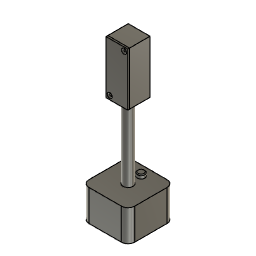
attiny85-traffic-light (Autodesk Fusion 360 design; units mm, degrees)
Autodesk Fusion 360 part; units mm, degrees
note: some values were not read from the file. Set by a fixed rule: which sketch regions a step uses.
sketch "Sketch1" plane through (0, 0, 0) normal (0, 1, 0) x (1, 0, 0)
  line L0 (0, 0) -> (17.5, 0)
  line L1 (17.5, 0) -> (17.5, -42.6)
  line L2 (17.5, -42.6) -> (0, -42.6)
  line L3 (0, -42.6) -> (0, 0)
  circle A0 centre (8.75, -21.3) radius 4.9
  line L4 (0, -21.3) -> (17.5, -21.3) construction
  circle A1 centre (8.75, -33.85) radius 4.9
  circle A2 centre (8.75, -8.75) radius 4.9
  line L5 (1.44, -1.44) -> (16.06, -1.44)
  line L6 (16.06, -1.44) -> (16.06, -41.16)
  line L7 (16.06, -41.16) -> (1.44, -41.16)
  line L8 (1.44, -41.16) -> (1.44, -1.44)
  circle A3 centre (14.5, -39.6) radius 3
  line L9 (11.5, -39.6) -> (11.5, -42.6)
  line L10 (14.5, -36.6) -> (17.5, -36.6)
  circle A4 centre (14.5, -39.6) radius 1.25
  circle A5 centre (3, -3) radius 3
  line L11 (6, -3) -> (6, 0)
  line L12 (3, -6) -> (0, -6)
  circle A6 centre (3, -3) radius 1.25
  circle A7 centre (14.5, -39.6) radius 1
  circle A8 centre (3, -3) radius 1
  line L13 (1.64, -1.64) -> (15.86, -1.64)
  line L14 (15.86, -1.64) -> (15.86, -40.96)
  line L15 (15.86, -40.96) -> (1.64, -40.96)
  line L16 (1.64, -40.96) -> (1.64, -1.64)
  dimension "d4" = 17.5
  dimension "d5" = 42.6
  dimension "d6" = 9.8
  dimension "d9" = 0
  dimension "d10" = 12.55
  dimension "d14" = 1.44
  dimension "d22" = 3
  dimension "d23" = 2.5
  dimension "d24" = 3
  dimension "d25" = 2.5
  dimension "d31" = 2
  dimension "d32" = 2
  dimension "d37" = 1.64
  constraint horizontal L0
  constraint vertical L1
  constraint horizontal L2
  constraint vertical L3
  constraint coincident L0.start L3.end
  constraint midpoint L3 L4.start
  constraint midpoint L1 L4.end
  constraint midpoint A0.centre L4
  constraint tangent L2 A3
  constraint tangent L1 A3
  constraint coincident A3 L9.start
  constraint coincident L2 L9.end
  constraint tangent A3 L9
  constraint perpendicular L2 L9
  constraint coincident A3 L10.start
  constraint coincident L1 L10.end
  constraint tangent A3 L10
  constraint perpendicular L1 L10
  constraint concentric A3 A4
  constraint tangent L3 A5
  constraint tangent L0 A5
  constraint coincident A5 L11.start
  constraint coincident L0 L11.end
  constraint tangent A5 L11
  constraint perpendicular L0 L11
  constraint coincident A5 L12.start
  constraint coincident L3 L12.end
  constraint tangent A5 L12
  constraint perpendicular L3 L12
  constraint concentric A5 A6
  constraint concentric A3 A7
  constraint concentric A6 A8
  measures "d4" distance of L0.start L0.end
  measures "d5" distance of L0.start L2.end
  measures "d6" diameter of A0
  measures "d22" radius of A3
  measures "d23" diameter of A4
  measures "d24" radius of A5
  measures "d25" diameter of A6
  measures "d31" diameter of A7
  measures "d32" diameter of A8
extrude "Extrude1" add sketch "Sketch1" along normal blind 4.44 contours L0 L5 A5 L11 | L0 L1 L5 L6 L10 L11 | L0 L3 A5 | L5 L8 A5 | L5 A5 L11 L13 | L5 L6 L10 L11 L13 L14 | L1 L6 A3 L10 | L5 L8 A5 L13 L16 | L3 L8 A5 L12 | A3 L9 L10 A5 L11 L12 L13 L14 L15 L16 | A5 L11 L13 | L6 L7 A3 | L1 L2 A3 | L6 A3 L10 L14 | A5 L13 L16 | L2 L3 L7 L8 L9 L12 | L8 A5 L12 L16 | L6 L7 A3 L14 L15 | L2 L7 A3 L9 | A3 L10 L14 | L7 L8 L9 L12 L15 L16 | A5 L12 L16 | A3 L14 L15 | L7 A3 L9 L15 | A3 L9 L15 | A4 | A6 | A7 | A8 makes body 1
extrude "Extrude2" add sketch "Sketch1" against normal blind 12.06 separate body contours L0 L5 A5 L11 | L0 L1 L5 L6 L10 L11 | L0 L3 A5 | L5 L8 A5 | L1 L6 A3 L10 | L3 L8 A5 L12 | L6 L7 A3 | L1 L2 A3 | L2 L3 L7 L8 L9 L12 | L2 L7 A3 L9 makes body 2
extrude "Extrude3" add sketch "Sketch1" against normal blind 11.26 separate body contours L5 A5 L11 L13 | L5 L8 A5 L13 L16 | A5 L11 L13 | L6 A3 L10 L14 | A5 L13 L16 | L8 A5 L12 L16 | L6 L7 A3 L14 L15 | A3 L10 L14 | A5 L12 L16 | A3 L14 L15 | L7 A3 L9 L15 | A3 L9 L15 makes body 3 at (13.3254, -7.5067, 40.0275) makes body 4 at (4.2438, -3.7533, 3.1245)
combine "Combine1" operation add target body 2 tool bodies 3 4
combine "Combine2" operation add target body 1 tool bodies 2
extrude "Extrude4" add sketch "Sketch1" against normal blind 1.44 from surface at -12.06 separate body contours L0 L5 A5 L11 | L0 L1 L5 L6 L10 L11 | L0 L3 A5 | L5 L8 A5 | L5 A5 L11 L13 | L5 L6 L10 L11 L13 L14 | L1 L6 A3 L10 | L5 L8 A5 L13 L16 | L3 L8 A5 L12 | A3 L9 L10 A5 L11 L12 L13 L14 L15 L16 | A5 L11 L13 | L6 L7 A3 | L1 L2 A3 | L6 A3 L10 L14 | A5 L13 L16 | L2 L3 L7 L8 L9 L12 | L8 A5 L12 L16 | L6 L7 A3 L14 L15 | L2 L7 A3 L9 | A3 L10 L14 | L7 L8 L9 L12 L15 L16 | A5 L12 L16 | A3 L14 L15 | L7 A3 L9 L15 | A3 L9 L15 | A0 | A1 | A2 | A4 | A6 makes body 5
extrude "Extrude5" add sketch "Sketch1" along normal blind 0.6 from surface at -12.06 contours A3 L9 L10 A5 L11 L12 L13 L14 L15 L16 | A5 L11 L13 | A5 L13 L16 | A3 L10 L14 | A5 L12 L16 | A3 L14 L15 | A3 L9 L15 | A0 | A1 | A2 | A4 | A6 bodies 5
chamfer "Chamfer1" distance 1 angle 45 2 edges at (13.5677, -13.5, 39.9616) (2.0677, -13.5, 3.3616) on bodies 5
sketch "Sketch2" plane through (0, 0, 0) normal (0, 0, 1) x (1, 0, 0)
  circle A0 centre (8.75, -4.53) radius 3
  line L0 (0, 0) -> (17.5, 0)
  line L1 (17.5, 0) -> (17.5, 4.44)
  line L2 (17.5, 4.44) -> (0, 4.44)
  line L3 (0, 4.44) -> (0, 0)
  line L4 (0, 0) -> (17.5, 0)
  line L5 (17.5, 0) -> (17.5, -13.5)
  line L6 (17.5, -13.5) -> (0, -13.5)
  line L7 (0, -13.5) -> (0, 0)
  line L8 (8.75, 4.44) -> (8.75, -13.5)
  circle A1 centre (8.75, -4.53) radius 4
  circle A2 centre (8.75, -4.53) radius 3.8
  line L9 (8.75, -0.53) -> (8.95, -0.53)
  line L10 (8.95, -0.53) -> (8.95, -8.53)
  line L11 (8.95, -8.53) -> (8.75, -8.53)
  line L12 (8.75, -8.53) -> (8.75, -0.53)
  line L13 (8.75, -0.53) -> (8.55, -0.53)
  line L14 (8.55, -0.53) -> (8.55, -8.53)
  line L15 (8.55, -8.53) -> (8.75, -8.53)
  line L16 (8.75, -8.53) -> (8.75, -0.53)
  line L17 (8.75, -4.53) -> (4.75, -4.53)
  line L18 (8.75, -4.53) -> (12.75, -4.53)
  line L19 (12.75, -4.63) -> (4.75, -4.63)
  line L20 (4.75, -4.63) -> (4.75, -4.43)
  line L21 (4.75, -4.43) -> (12.75, -4.43)
  line L22 (12.75, -4.43) -> (12.75, -4.63)
  line L23 (12.75, -4.63) -> (4.75, -4.43) construction
  line L24 (4.75, -4.63) -> (12.75, -4.43) construction
  point P0 (8.75, -4.53)
  dimension "d41" = 6
  dimension "d42" = 17.5
  dimension "d43" = 4.44
  dimension "d44" = 17.5
  dimension "d45" = 13.5
  dimension "d46" = 1
  dimension "d52" = 0.8
  dimension "d53" = 0.2
  dimension "d54" = 8
  dimension "d124" = 0.2
  dimension "d125" = 8
  dimension "d126" = 8
  dimension "d127" = 0.2
  constraint horizontal L0
  constraint vertical L1
  constraint horizontal L2
  constraint vertical L3
  constraint coincident L0.start L3.end
  constraint horizontal L4
  constraint vertical L5
  constraint horizontal L6
  constraint vertical L7
  constraint midpoint L2 L8.start
  constraint midpoint L6 L8.end
  constraint midpoint P0 L8
  constraint horizontal L9
  constraint vertical L10
  constraint horizontal L11
  constraint vertical L12
  constraint coincident L8 L9.start
  constraint coincident A1 L9.start
  constraint horizontal L13
  constraint vertical L14
  constraint horizontal L15
  constraint vertical L16
  constraint coincident P0 A0.centre
  constraint coincident A1 L17.end
  constraint horizontal L17
  constraint coincident A1 L18.end
  constraint parallel L17 L18
  constraint horizontal L19
  constraint perpendicular L19 L20
  constraint parallel L19 L21
  constraint parallel L20 L22
  constraint coincident L23 P0
  constraint coincident L24 P0
  measures "d41" diameter of A0
  measures "d42" distance of L0.start L0.end
  measures "d43" distance of L0.start L2.end
  measures "d44" distance of L0.start L0.end
  measures "d45" distance of L0.start L6.end
  measures "d53" distance of L9.start L9.end
  measures "d54" distance of L9.start L11.end
  measures "d124" distance of L9.start L13.end
  measures "d125" distance of L9.start L11.end
  measures "d126" distance of L20.end L21.end
  measures "d127" distance of L19.end L20.end
extrude "Extrude6" add sketch "Sketch2" against normal blind 60 separate body contours A0 A2 L18 L19 | A0 A2 L18 L21 | A0 A2 L10 L21 | A0 A2 L10 L19 | A1 A2 L18 L19 L22 | A1 A2 L18 L21 L22 | A0 L8 A2 L10 L12 L16 | A1 A2 L10 L21 | A0 L8 A2 L10 L12 L16 | A1 A2 L10 L19 | A0 L8 A2 L12 L14 L16 | L8 A1 A2 L10 L12 L16 | A0 L8 A2 L12 L14 L16 | L8 A1 A2 L10 L12 L16 | A0 A2 L14 L21 | L8 A1 A2 L12 L14 L16 | A0 A2 L14 L19 | L8 A1 A2 L12 L14 L16 | A0 A2 L17 L21 | A0 A2 L17 L19 | A1 A2 L14 L21 | A1 A2 L14 L19 | A1 A2 L17 L20 L21 | A1 A2 L17 L19 L20 makes body 6
extrude "Extrude7" cut sketch "Sketch2" along normal blind 1.44 contours A0 L10 L18 L21 | A0 A2 L18 L19 | A0 A2 L18 L21 | A0 L10 L18 L19 | A0 L10 L21 | A0 A2 L10 L21 | A0 A2 L10 L19 | A0 L10 L19 | A1 A2 L18 L19 L22 | A1 A2 L18 L21 L22 | L8 L10 L12 L16 L18 L21 | L8 L10 L12 L16 L18 L19 | A0 L8 L10 L12 L16 L21 | A0 L8 A2 L10 L12 L16 | A1 A2 L10 L21 | A0 L8 A2 L10 L12 L16 | A0 L8 L10 L12 L16 L19 | A1 A2 L10 L19 | L8 L12 L14 L16 L17 L21 | L8 L12 L14 L16 L17 L19 | A0 L8 L12 L14 L16 L21 | L8 A1 A2 L10 L12 L16 | A0 L8 L12 L14 L16 L19 | L8 A1 A2 L10 L12 L16 | A0 L14 L17 L21 | A0 L14 L17 L19 | A0 L14 L21 | A0 L14 L19 bodies 1
extrude "Extrude8" add sketch "Sketch2" along normal blind 1.8 contours A0 A2 L18 L19 | A0 A2 L18 L21 | A0 A2 L10 L21 | A0 A2 L10 L19 bodies 6
ref_plane "WorkPlane1" through (0, 0, -83.68) normal (0, 0, 1) x (1, 0, 0)
sketch "Sketch3" plane through (0, 0, -83.68) normal (0, 0, 1) x (1, 0, 0)
  line L0 (0, 0) -> (8.75, 0) construction
  line L1 (8.75, 0) -> (8.75, -4.53) construction
  line L2 (8.75, -4.53) -> (0, -4.53) construction
  line L3 (0, -4.53) -> (0, 0) construction
  line L4 (21.75, 12.47) -> (-4.25, 12.47)
  line L5 (-8.25, 8.47) -> (-8.25, -17.53)
  line L6 (-4.25, -21.53) -> (21.75, -21.53)
  line L7 (25.75, -17.53) -> (25.75, 8.47)
  line L8 (25.75, 12.47) -> (-8.25, -21.53) construction
  line L9 (-8.25, 12.47) -> (25.75, -21.53) construction
  arc A0 (-8.25, -17.53) -> (-4.25, -21.53) centre (-4.25, -17.53) ccw
  arc A1 (21.75, -21.53) -> (25.75, -17.53) centre (21.75, -17.53) ccw
  arc A2 (25.75, 8.47) -> (21.75, 12.47) centre (21.75, 8.47) ccw
  arc A3 (-4.25, 12.47) -> (-8.25, 8.47) centre (-4.25, 8.47) ccw
  line L10 (-9.69, 8.47) -> (-9.69, -17.53)
  arc A4 (-9.69, -17.53) -> (-4.25, -22.97) centre (-4.25, -17.53) ccw
  line L11 (-4.25, -22.97) -> (21.75, -22.97)
  arc A5 (21.75, -22.97) -> (27.19, -17.53) centre (21.75, -17.53) ccw
  line L12 (27.19, -17.53) -> (27.19, 8.47)
  arc A6 (27.19, 8.47) -> (21.75, 13.91) centre (21.75, 8.47) ccw
  line L13 (21.75, 13.91) -> (-4.25, 13.91)
  arc A7 (-4.25, 13.91) -> (-9.69, 8.47) centre (-4.25, 8.47) ccw
  line L14 (-8.05, 8.47) -> (-8.05, -17.53)
  arc A8 (-8.05, -17.53) -> (-4.25, -21.33) centre (-4.25, -17.53) ccw
  line L15 (-4.25, -21.33) -> (21.75, -21.33)
  arc A9 (21.75, -21.33) -> (25.55, -17.53) centre (21.75, -17.53) ccw
  line L16 (25.55, -17.53) -> (25.55, 8.47)
  arc A10 (25.55, 8.47) -> (21.75, 12.27) centre (21.75, 8.47) ccw
  line L17 (21.75, 12.27) -> (-4.25, 12.27)
  arc A11 (-4.25, 12.27) -> (-8.05, 8.47) centre (-4.25, 8.47) ccw
  line L18 (25.75, -4.53) -> (-8.25, -4.53) construction
  line L19 (8.75, -4.53) -> (12.75, -4.53) construction
  circle A12 centre (12.75, -4.53) radius 11
  line L20 (8.75, -4.53) -> (-3.25, -4.53) construction
  line L21 (-0.25, -14.53) -> (-6.25, -14.53)
  line L22 (-6.25, -14.53) -> (-6.25, 5.47)
  line L23 (-6.25, 5.47) -> (-0.25, 5.47)
  line L24 (-0.25, 5.47) -> (-0.25, -14.53)
  line L25 (-0.25, -14.53) -> (-6.25, 5.47) construction
  line L26 (-6.25, -14.53) -> (-0.25, 5.47) construction
  line L27 (-6.25, -10.43) -> (-0.25, -10.43)
  line L28 (-0.25, -10.43) -> (-0.25, 1.37)
  line L29 (-0.25, 1.37) -> (-6.25, 1.37)
  line L30 (-6.25, 1.37) -> (-6.25, -10.43)
  line L31 (-6.25, -10.43) -> (-0.25, 1.37) construction
  line L32 (-0.25, -10.43) -> (-6.25, 1.37) construction
  line L33 (1.75, -15.53) -> (23.75, -15.53) construction
  line L34 (23.75, -15.53) -> (23.75, 6.47) construction
  line L35 (23.75, 6.47) -> (1.75, 6.47) construction
  line L36 (1.75, 6.47) -> (1.75, -15.53) construction
  line L37 (1.75, -15.53) -> (23.75, 6.47) construction
  line L38 (23.75, -15.53) -> (1.75, 6.47) construction
  line L39 (4.9718, 3.2482) -> (8.1937, 6.47) construction
  circle A13 centre (3.6373, 4.5827) radius 1.8873 construction
  line L40 (4.9718, -12.3082) -> (8.1937, -15.53) construction
  circle A14 centre (3.6373, -13.6427) radius 1.8873 construction
  circle A15 centre (12.75, -4.53) radius 4
  circle A16 centre (3.6373, 4.5827) radius 0.6
  circle A17 centre (3.6373, -13.6427) radius 0.6
  line L41 (9.2756, -2.548) -> (3.1161, -13.3454)
  line L42 (3.9346, -14.1639) -> (14.732, -8.0044)
  line L43 (3.9346, 5.1039) -> (14.732, -1.0556)
  line L44 (3.1161, 4.2854) -> (9.2756, -6.512)
  line L45 (-4.95, -7.63) -> (-1.55, -7.63)
  line L46 (-1.55, -7.63) -> (-1.55, -1.43)
  line L47 (-1.55, -1.43) -> (-4.95, -1.43)
  line L48 (-4.95, -1.43) -> (-4.95, -7.63)
  line L49 (-4.95, -7.63) -> (-1.55, -1.43) construction
  line L50 (-1.55, -7.63) -> (-4.95, -1.43) construction
  circle A18 centre (-4.25, -17.53) radius 1.25
  circle A19 centre (-4.25, -17.53) radius 2.2
  circle A20 centre (21.75, 8.47) radius 1.25
  circle A21 centre (21.75, 8.47) radius 2.2
  circle A22 centre (-4.25, -17.53) radius 1.9
  circle A23 centre (21.75, 8.47) radius 1.9
  line L51 (-3.25, -4.53) -> (-3.25, 3.47) construction
  line L52 (-3.25, -4.53) -> (-3.25, -12.53) construction
  circle A24 centre (-3.25, -12.53) radius 1
  circle A25 centre (-3.25, 3.47) radius 1
  line L53 (8.75, -4.53) -> (19.25, -4.53) construction
  circle A26 centre (19.25, -4.53) radius 3
  line L54 (25.75, 5.97) -> (-8.25, 5.97)
  line L55 (-8.25, 5.97) -> (-8.25, -15.03)
  line L56 (-8.25, -15.03) -> (25.75, -15.03)
  line L57 (25.75, -15.03) -> (25.75, 5.97)
  line L58 (25.75, 5.97) -> (-8.25, -15.03) construction
  line L59 (-8.25, 5.97) -> (25.75, -15.03) construction
  line L60 (1.75, -17.53) -> (15.75, -17.53)
  line L61 (15.75, -17.53) -> (15.75, 8.47)
  line L62 (15.75, 8.47) -> (1.75, 8.47)
  line L63 (1.75, 8.47) -> (1.75, -17.53)
  line L64 (1.75, -17.53) -> (15.75, 8.47)
  line L65 (15.75, -17.53) -> (1.75, 8.47)
  circle A27 centre (19.25, -4.53) radius 2.9
  circle A28 centre (19.25, -4.53) radius 4.5
  point P0 (8.75, -4.53)
  point P1 (-3.25, -4.53)
  point P2 (-3.25, -4.53)
  point P3 (12.75, -4.53)
  point P4 (-3.25, -4.53)
  point P5 (8.75, -4.53)
  point P6 (8.75, -4.53)
  dimension "d57" = 8.75
  dimension "d58" = 4.53
  dimension "d59" = 34
  dimension "d60" = 34
  dimension "d61" = 4
  dimension "d62" = 1.44
  dimension "d64" = 4
  dimension "d65" = 22
  dimension "d66" = 12
  dimension "d67" = 6
  dimension "d68" = 20
  dimension "d69" = 6
  dimension "d70" = 11.8
  dimension "d71" = 22
  dimension "d72" = 22
  dimension "d73" = 8
  dimension "d74" = 1.2
  dimension "d75" = 1.2
  dimension "d76" = 3.4
  dimension "d77" = 6.2
  dimension "d80" = 2.5
  dimension "d81" = 4.4
  dimension "d82" = 2.5
  dimension "d83" = 4.4
  dimension "d87" = 3.8
  dimension "d88" = 3.8
  dimension "d99" = 8
  dimension "d100" = 8
  dimension "d101" = 2
  dimension "d102" = 2
  dimension "d114" = 10.5
  dimension "d115" = 6
  dimension "d116" = 34
  dimension "d117" = 21
  dimension "d135" = 14
  dimension "d136" = 26
  dimension "d140" = 5.8
  dimension "d141" = 9
  constraint horizontal L0
  constraint vertical L1
  constraint horizontal L2
  constraint vertical L3
  constraint coincident L0.start L3.end
  constraint horizontal L4
  constraint perpendicular L4 L5
  constraint parallel L4 L6
  constraint parallel L5 L7
  constraint coincident L8 P6
  constraint coincident L9 P6
  constraint coincident P6 P5
  constraint coincident L8.end L5
  constraint coincident L8.end L6
  constraint tangent L5 A0
  constraint tangent L6 A0
  constraint coincident L9.end L6
  constraint coincident L9.end L7
  constraint tangent L6 A1
  constraint tangent L7 A1
  constraint equal A0 A1
  constraint coincident L8.start L7
  constraint coincident L8.start L4
  constraint tangent L7 A2
  constraint tangent L4 A2
  constraint equal A0 A2
  constraint coincident L9.start L5
  constraint coincident L9.start L4
  constraint tangent L5 A3
  constraint tangent L4 A3
  constraint equal A0 A3
  constraint midpoint L7 L18.start
  constraint midpoint L5 L18.end
  constraint parallel L18 L19
  constraint coincident P3 L19.end
  constraint perpendicular L3 L20
  constraint horizontal L21
  constraint perpendicular L21 L22
  constraint parallel L21 L23
  constraint parallel L22 L24
  constraint coincident L25 P4
  constraint coincident L26 P4
  constraint coincident P4 P2
  constraint horizontal L27
  constraint perpendicular L27 L28
  constraint parallel L27 L29
  constraint parallel L28 L30
  constraint coincident L31 P4
  constraint coincident L32 P4
  constraint horizontal L33
  constraint perpendicular L33 L34
  constraint parallel L33 L35
  constraint parallel L34 L36
  constraint coincident L37 P3
  constraint coincident L38 P3
  constraint coincident A12 L39.start
  constraint coincident L38 L39.start
  constraint coincident L35 L39.end
  constraint tangent A12 L39
  constraint tangent L39 A13
  constraint tangent L35 A13
  constraint tangent L36 A13
  constraint coincident A12 L40.start
  constraint coincident L37 L40.start
  constraint coincident L33 L40.end
  constraint tangent A12 L40
  constraint tangent L36 A14
  constraint tangent L33 A14
  constraint tangent L40 A14
  constraint concentric A12 A15
  constraint concentric A13 A16
  constraint concentric A14 A17
  constraint coincident A15 L41.start
  constraint coincident A17 L41.end
  constraint tangent A17 L41
  constraint tangent A15 L41
  constraint coincident A17 L42.start
  constraint coincident A15 L42.end
  constraint tangent A15 L42
  constraint tangent A17 L42
  constraint coincident A16 L43.start
  constraint coincident A15 L43.end
  constraint tangent A15 L43
  constraint tangent A16 L43
  constraint coincident A16 L44.start
  constraint coincident A15 L44.end
  constraint tangent A16 L44
  constraint tangent A15 L44
  constraint horizontal L45
  constraint perpendicular L45 L46
  constraint parallel L45 L47
  constraint parallel L46 L48
  constraint coincident L49 P4
  constraint coincident L50 P4
  constraint concentric A0 A18
  constraint concentric A0 A19
  constraint concentric A2 A20
  constraint concentric A2 A21
  constraint concentric A0 A22
  constraint concentric A2 A23
  constraint perpendicular L29 L51
  constraint perpendicular L27 L52
  constraint coincident L52.end A24.centre
  constraint coincident L51.end A25.centre
  constraint perpendicular L3 L53
  constraint coincident L53.end A26.centre
  constraint horizontal L54
  constraint perpendicular L54 L55
  constraint parallel L54 L56
  constraint parallel L55 L57
  constraint coincident L58 P6
  constraint coincident L59 P6
  constraint horizontal L60
  constraint perpendicular L60 L61
  constraint parallel L60 L62
  constraint parallel L61 L63
  constraint coincident L64 P6
  constraint coincident L65 P6
  constraint concentric A26 A27
  constraint concentric A26 A28
  measures "d57" distance of L0.start L0.end
  measures "d58" distance of L0.start L2.end
  measures "d59" distance of L8.end L9.end
  measures "d60" distance of L9.start L8.end
  measures "d61" radius of A0
  measures "d64" distance of P6 P3
  measures "d65" diameter of A12
  measures "d66" distance of P6 P4
  measures "d67" distance of L22.end L23.end
  measures "d68" distance of L21.end L22.end
  measures "d69" distance of L28.end L29.end
  measures "d70" distance of L27.end L28.end
  measures "d71" distance of L34.end L35.end
  measures "d72" distance of L33.end L34.end
  measures "d73" diameter of A15
  measures "d74" diameter of A16
  measures "d75" diameter of A17
  measures "d76" distance of L46.end L47.end
  measures "d77" distance of L45.end L46.end
  measures "d80" diameter of A18
  measures "d81" diameter of A19
  measures "d82" diameter of A20
  measures "d83" diameter of A21
  measures "d87" diameter of A22
  measures "d88" diameter of A23
  measures "d99" distance of P4 L51.end
  measures "d100" distance of P4 L52.end
  measures "d101" diameter of A24
  measures "d102" diameter of A25
  measures "d114" distance of P6 L53.end
  measures "d115" diameter of A26
  measures "d116" distance of L55.end L56.end
  measures "d117" distance of L54.end L55.end
  measures "d135" distance of L61.end L62.end
  measures "d136" distance of L60.end L61.end
  measures "d140" diameter of A27
  measures "d141" diameter of A28
extrude "Extrude9" add sketch "Sketch3" against normal blind 1.44 separate body contours L14 L16 A10 L17 A11 A12 L54 L61 L62 L63 | L16 A12 L54 L56 | L14 L54 L56 L63 | L14 A8 L15 A9 L16 A12 L56 L60 L61 L63 | A12 L54 L61 | A12 L54 L61 A28 | L54 L63 L65 | A12 A16 L44 L54 L63 L65 | A12 L56 L61 A28 | A12 L56 L61 | A15 A26 L61 A28 | A12 L54 L61 L64 | A12 L61 L64 | A15 L43 L54 L61 L64 A28 | A12 A17 L41 L56 L63 L64 | L56 L63 L64 | A12 L54 L62 L64 L65 | A12 A16 L43 L54 L65 | A12 L41 L44 | A12 L61 L65 | A12 L56 L61 L65 | A15 L42 L56 L61 L65 A28 | A15 L61 A28 | A15 L61 A28 | A12 L54 L64 | A12 L43 L54 L64 | A12 A17 L42 L56 L64 | A12 L56 L60 L64 L65 | A16 L65 | A16 L65 | A12 A16 L44 L65 | A12 L41 L44 L65 | A12 L41 L44 L64 | A12 A17 L41 L64 | A12 L56 L65 | A12 L42 L56 L65 | A15 L61 A28 | A15 A26 L61 | A15 L64 L65 A28 | A12 A15 L41 L43 L64 L65 | A15 L43 L64 | A17 L64 | A17 L64 | A12 A16 L43 L65 | L41 L44 L64 L65 | A12 A15 L42 L44 L64 L65 | A12 A17 L42 L64 | A15 L42 L65 | A15 A26 A27 | A15 A26 A27 | A15 L64 | A15 L41 L65 | A15 L44 L64 | A15 L65 | A15 A27 | A15 A27 | L21 L22 L24 L27 | L22 L24 L27 L28 L29 L30 | L22 L23 L24 L29 | A19 | A21 | A22 | A23 | A24 | A25 makes body 7
chamfer "Chamfer2" distance 1 angle 45 2 edges at (20.5846, 8.018, -85.12) (-5.4154, -17.982, -85.12) on bodies 7
extrude "Extrude10" add sketch "Sketch3" along normal blind 8 separate body contours L14 L16 A10 L17 A11 A12 L54 L61 L62 L63 | L16 A12 L54 L56 | L14 L54 L56 L63 | L14 A8 L15 A9 L16 A12 L56 L60 L61 L63 | L54 L63 L65 | A12 A16 L44 L54 L63 L65 | A12 L61 L64 | A12 A17 L41 L56 L63 L64 | L56 L63 L64 | A12 L54 L62 L64 L65 | A12 A16 L43 L54 L65 | A12 L61 L65 | A12 A17 L42 L56 L64 | A12 L56 L60 L64 L65 | L21 L22 L24 L27 | L22 L23 L24 L29 | A19 | A21 makes body 8
extrude "Extrude11" add sketch "Sketch3" along normal blind 1.44 from surface at 8 contours L14 L16 A10 L17 A11 A12 L54 L61 L62 L63 | L16 A12 L54 L56 | L14 L54 L56 L63 | L14 A8 L15 A9 L16 A12 L56 L60 L61 L63 | A12 L54 L61 | A12 L54 L61 A28 | L54 L63 L65 | A12 A16 L44 L54 L63 L65 | A12 L56 L61 A28 | A12 L56 L61 | A15 A26 L61 A28 | A12 L54 L61 L64 | A12 L61 L64 | A15 L43 L54 L61 L64 A28 | A12 A17 L41 L56 L63 L64 | L56 L63 L64 | A12 L54 L62 L64 L65 | A12 A16 L43 L54 L65 | A12 L41 L44 | A12 L61 L65 | A12 L56 L61 L65 | A15 L42 L56 L61 L65 A28 | A15 L61 A28 | A15 L61 A28 | A12 L54 L64 | A12 L43 L54 L64 | A12 A17 L42 L56 L64 | A12 L56 L60 L64 L65 | A12 A16 L44 L65 | A12 L41 L44 L65 | A12 L41 L44 L64 | A12 A17 L41 L64 | A12 L56 L65 | A12 L42 L56 L65 | A15 L61 A28 | A15 A26 L61 | A15 L64 L65 A28 | A12 A15 L41 L43 L64 L65 | A15 L43 L64 | A12 A16 L43 L65 | L41 L44 L64 L65 | A12 A15 L42 L44 L64 L65 | A12 A17 L42 L64 | A15 L42 L65 | A15 A26 A27 | A15 A26 A27 | A15 L64 | A15 L41 L65 | A15 L44 L64 | A15 L65 | A15 A27 | A15 A27 | L21 L22 L24 L27 | L22 L23 L24 L29 | A19 | A21 bodies 8
extrude "Extrude12" cut sketch "Sketch3" along normal blind 5.06 contours L21 L22 L24 L27 | L22 L23 L24 L29 | A24 | A25 bodies 8
extrude "Extrude13" add sketch "Sketch3" against normal blind 0.6 from surface at 8 contours A12 L54 L61 | A12 L54 L61 A28 | A12 L56 L61 A28 | A12 L56 L61 | A15 A26 L61 A28 | A12 L54 L61 L64 | A15 L43 L54 L61 L64 A28 | A12 L41 L44 | A12 L56 L61 L65 | A15 L42 L56 L61 L65 A28 | A15 L61 A28 | A15 L61 A28 | A12 L54 L64 | A12 L43 L54 L64 | A12 L56 L65 | A12 L42 L56 L65 | A15 A26 A27 | A15 A27 picked at (15.7414, -1.7733) picked at (15.7414, -7.2867) picked at (18.5835, -7.3815) picked at (20.34, -4.3912) bodies 8
extrude "Extrude14" add sketch "Sketch3" along normal blind 23.68 separate body contours L10 A4 L11 A5 L12 A6 L13 A7 makes body 9
extrude "Extrude15" add sketch "Sketch3" 1 faces at (26.71, -1.03, -83.68) against normal blind 1.44 from surface at 23.68 contours L4 L5 L7 A2 A3 L14 L16 A10 L17 A11 L54 | L7 L16 L54 L56 L57 | L5 L14 L54 L55 L56 | L5 L6 L7 A0 A1 L14 A8 L15 A9 L16 L56 | L14 L16 A10 L17 A11 A12 L54 L61 L62 L63 | L16 A12 L54 L56 | L14 L54 L56 L63 | L14 A8 L15 A9 L16 A12 L56 L60 L61 L63 | A12 L54 L61 | A12 L54 L61 A28 | L54 L63 L65 | A12 A16 L44 L54 L63 L65 | A12 L56 L61 A28 | A12 L56 L61 | A15 A26 L61 A28 | A12 L54 L61 L64 | A12 L61 L64 | A15 L43 L54 L61 L64 A28 | A12 A17 L41 L56 L63 L64 | L56 L63 L64 | A12 L54 L62 L64 L65 | A12 A16 L43 L54 L65 | A12 L41 L44 | A12 L61 L65 | A12 L56 L61 L65 | A15 L42 L56 L61 L65 A28 | A15 L61 A28 | A15 L61 A28 | A12 L54 L64 | A12 L43 L54 L64 | A12 A17 L42 L56 L64 | A12 L56 L60 L64 L65 | A16 L65 | A16 L65 | A12 A16 L44 L65 | A12 L41 L44 L65 | A12 L41 L44 L64 | A12 A17 L41 L64 | A12 L56 L65 | A12 L42 L56 L65 | A15 L61 A28 | A15 A26 L61 | A15 L64 L65 A28 | A12 A15 L41 L43 L64 L65 | A15 L43 L64 | A17 L64 | A17 L64 | A12 A16 L43 L65 | L41 L44 L64 L65 | A12 A15 L42 L44 L64 L65 | A12 A17 L42 L64 | A15 L42 L65 | A15 A26 A27 | A15 A26 A27 | A15 L64 | A15 L41 L65 | A15 L44 L64 | A15 L65 | A15 A27 | A15 A27 | L10 A4 L11 A5 L12 A6 L13 A7 | L21 L22 L24 L27 | L22 L24 L27 L28 L29 L30 | L22 L23 L24 L29 | L45 L46 L47 L48 | A18 | A19 | A20 | A21 | A22 | A23 | A24 | A25 on bodies 9 bodies 9
extrude "Extrude16" add sketch "Sketch3" against normal blind 1.44 contours L10 A4 L11 A5 L12 A6 L13 A7 bodies 9
extrude "Extrude17" cut sketch "Sketch3" along normal blind 50 contours A15 A26 A27 | A15 A26 A27 | A15 A27 | A15 A27 bodies 9
extrude "Extrude18" add sketch "Sketch3" along normal blind 14.04 from surface at 9.64 contours L4 L5 L7 A2 A3 L14 L16 A10 L17 A11 L54 | L5 L6 L7 A0 A1 L14 A8 L15 A9 L16 L56 | L14 L16 A10 L17 A11 A12 L54 L61 L62 L63 | L14 A8 L15 A9 L16 A12 L56 L60 L61 L63 | A12 L54 L61 | L54 L63 L65 | A12 L56 L61 | A12 L54 L61 L64 | A12 L61 L64 | L56 L63 L64 | A12 L54 L62 L64 L65 | A12 L61 L65 | A12 L56 L61 L65 | A12 L54 L64 | A12 L56 L60 L64 L65 | A12 L56 L65 | A19 | A21 bodies 9
extrude "Extrude19" add sketch "Sketch2" against normal blind 1.8 from surface at -60 contours A0 A2 L14 L21 | A0 A2 L14 L19 | A0 A2 L17 L21 | A0 A2 L17 L19 bodies 6
extrude "Extrude20" cut sketch "Sketch2" against normal blind 1.44 from surface at -60 contours A0 L10 L18 L21 | A0 A2 L18 L21 | A0 L10 L18 L19 | A0 L10 L21 | A0 A2 L10 L21 | A0 L10 L19 | A1 A2 L18 L21 L22 | L8 L10 L12 L16 L18 L21 | L8 L10 L12 L16 L18 L19 | A0 L8 L10 L12 L16 L21 | A0 L8 A2 L10 L12 L16 | A1 A2 L10 L21 | A0 L8 L10 L12 L16 L19 | L8 L12 L14 L16 L17 L21 | L8 L12 L14 L16 L17 L19 | A0 L8 L12 L14 L16 L21 | A0 L8 A2 L12 L14 L16 | L8 A1 A2 L10 L12 L16 | A0 L8 L12 L14 L16 L19 | A0 L14 L17 L21 | A0 L14 L17 L19 | A0 L14 L21 | A0 A2 L14 L21 | L8 A1 A2 L12 L14 L16 | A0 L14 L19 | A0 A2 L17 L21 | A1 A2 L14 L21 | A1 A2 L17 L20 L21 picked at (8.8612, -1.2653) picked at (8.6388, -1.2653) picked at (8.9278, -0.6675) picked at (8.5722, -0.6675) bodies 9
extrude "Extrude21" cut sketch "Sketch3" along normal blind 0.48 from surface at -1.44 contours L54 L63 L65 | A12 A16 L44 L54 L63 L65 | A12 L54 L61 L64 | A12 L61 L64 | A15 L43 L54 L61 L64 A28 | A12 A17 L41 L56 L63 L64 | L56 L63 L64 | A12 L54 L62 L64 L65 | A12 A16 L43 L54 L65 | A12 L41 L44 | A12 L61 L65 | A12 L56 L61 L65 | A15 L42 L56 L61 L65 A28 | A15 L61 A28 | A15 L61 A28 | A12 L54 L64 | A12 L43 L54 L64 | A12 A17 L42 L56 L64 | A12 L56 L60 L64 L65 | A16 L65 | A16 L65 | A12 A16 L44 L65 | A12 L41 L44 L65 | A12 L41 L44 L64 | A12 A17 L41 L64 | A12 L56 L65 | A12 L42 L56 L65 | A15 L61 A28 | A15 L64 L65 A28 | A12 A15 L41 L43 L64 L65 | A15 L43 L64 | A17 L64 | A17 L64 | A12 A16 L43 L65 | L41 L44 L64 L65 | A12 A15 L42 L44 L64 L65 | A12 A17 L42 L64 | A15 L42 L65 | A15 L64 | A15 L41 L65 | A15 L44 L64 | A15 L65 bodies 7
extrude "Extrude22" add sketch "Sketch3" along normal blind 3 and the other way blind 6.3 from surface at 23.68 separate body contours A15 A26 A27 | A15 A26 A27 | A15 A27 | A15 A27 makes body 10
extrude "Extrude23" add sketch "Sketch3" along normal blind 4.26 from surface at 17.38 contours A15 A26 L61 A28 | A15 L61 A28 | A15 A26 L61 | A15 A26 A27 | A15 A26 A27 | A15 A27 | A15 A27 picked at (15.4206, -4.6386) bodies 10
fillet "Fillet1" radius 0.6 1 faces at (17.8211, -4.6127, -57) on bodies 10
move_body "Move1" bodies 9 8 7 10 to x (0, 1, 0) y (-1, 0, 0) z (0, 0, 1) at (4.22, -13.28, 0)
equation "lamp_radius = 4.9 mm"
equation "lamp_margin_inter = 2.75 mm"
equation "lamp_margin_outer = 3.85 mm"
equation "d4 = 2 * lamp_radius + 2 * lamp_margin_outer"
equation "d5 = 3 * 2 * lamp_radius + 2 * lamp_margin_inter + 2 * lamp_margin_outer"
equation "d6 = 2 * lamp_radius"
equation "d10 = 2 * lamp_radius + lamp_margin_inter"
equation "d11 = led_socket_depth"
equation "wall_thickness = 1.44 mm"
equation "d14 = wall_thickness"
equation "led_socket_depth = 4.44 mm"
equation "led_base_depth = 1.98 mm"
equation "d17 = -( led_base_depth + lamp_inner_space )"
equation "lamp_inner_space = 10.08 mm"
equation "lamp_screw_margin = 6 mm"
equation "lamp_insert_diam = 2.5 mm"
equation "d22 = lamp_screw_margin / 2"
equation "d23 = lamp_insert_diam"
equation "d24 = lamp_screw_margin / 2"
equation "d25 = lamp_insert_diam"
equation "d26 = -( lamp_inner_space + led_base_depth - lamp_backface_inset - pla_expansion )"
equation "lamp_backface_inset = 0.6 mm"
equation "pla_expansion = 0.2 mm"
equation "lamp_screw_diam = 2 mm"
equation "d31 = lamp_screw_diam"
equation "d32 = lamp_screw_diam"
equation "d33 = -( lamp_inner_space + led_base_depth )"
equation "d34 = -wall_thickness"
equation "d36 = ( 4 mm - lamp_screw_diam ) / 2"
equation "d37 = pla_expansion + wall_thickness"
equation "d38 = -( lamp_inner_space + led_base_depth )"
equation "d39 = lamp_backface_inset"
equation "d42 = 2 * lamp_radius + 2 * lamp_margin_outer"
equation "d43 = led_socket_depth"
equation "d44 = 2 * lamp_radius + 2 * lamp_margin_outer"
equation "d45 = lamp_inner_space + wall_thickness + led_base_depth"
equation "pole_height = 60 mm"
equation "d48 = -pole_height"
equation "d50 = wall_thickness"
equation "d52 = 1.00 mm - pla_expansion"
equation "d55 = 1.25 * wall_thickness"
equation "d57 = lamp_radius + lamp_margin_outer"
equation "d58 = ( lamp_inner_space + led_base_depth + wall_thickness + led_socket_depth ) / 2 - led_socket_depth"
equation "d62 = wall_thickness"
equation "d63 = -pla_expansion"
equation "switch_height = 6 mm"
equation "battery_height = 3.2 mm"
equation "d84 = -wall_thickness"
equation "d92 = wall_thickness"
equation "d94 = 6.5 mm - wall_thickness"
equation "pcb_height = 12 mm"
equation "d104 = 8 mm + wall_thickness + 0.8 mm + pcb_height + wall_thickness"
equation "base_height = 8 mm + wall_thickness + 0.8 mm + pcb_height + wall_thickness"
equation "d107 = base_height"
equation "d108 = -wall_thickness"
equation "d110 = -pole_height - base_height"
equation "d111 = -wall_thickness"
equation "d120 = base_inset_from_bottom - wall_thickness - 0.6 mm"
equation "d121 = pcb_height + wall_thickness + 0.6 mm"
equation "base_inset_from_bottom = 8 mm + wall_thickness + 0.8 mm + wall_thickness"
equation "d128 = -pole_height"
equation "d129 = -1.25 * wall_thickness"
equation "d131 = -pole_height"
equation "d132 = -wall_thickness"
equation "d137 = -wall_thickness"
equation "button_max_depth = 6.3 mm"
equation "button_travel = 0.6 mm"
equation "button_outer_height = 3 mm"
equation "d145 = base_height"
equation "d146 = button_outer_height"
equation "d148 = button_max_depth"
equation "d151 = button_max_depth - wall_thickness - button_travel"
named bodies: "Front", "Sides", "Back", "Pole", "Battery cover", "Battery holder", "Base", "Button"
